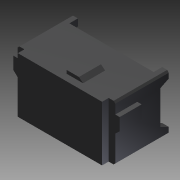
# Autodesk Inventor part: AS11CHright12
Saved by Autodesk Inventor 2011 SP1 (Build 150282100, 282)
## iProperties
Created: 2018-06-01
Part Number: AS11CHright12
Catalog Web Link: www.cadenas.de
Description: AS - Series - Body 1_2 for Poles 1 - Right Angle-
Vendor: NKKSWITCHES
Document SubType Name: Modeling
Designer: psAdmin
Manufacturer: NKKSWITCHES
Mass: 0.217145 g
Surface Area: 2.37031 cm^2
Volume: 0.217145 cm^3
Density: 1 g/cm^3
Category: PARTsolutions
Company: NKKSWITCHES
Title: AS11CHright12
Author: Cadenas PARTsolutions
PSOL_IDENT_0: {$CADENAS_DATA\23d-libs\nkkswitches\slides\as\parts\as_body_right1_2.prj},231 {VTYP=3D},{NB=AS11CHri
PSOL_IDENT_1: ght12},{LINA=AS11CHright12},{NN=AS - Series - Body 1_2 for Poles 1 - Right Angle},{DATE=11.10.2017 1
PSOL_IDENT_2: 0:53:50},{GEOMDATE=16.12.2008 13:32:00},{VERSION=},{LINEID=10},{LINESUBID=-1},{WBVAR=PLS,CRCTS,ACTU,
PSOL_IDENT_3: TRMNLS}  {NB=AS11CHright12},{LINA=AS11CHright12},{KT=DUMMY},{PN=AS11CH},{SRS=AS},{PLS=1},{CRCTS=1},{
PSOL_IDENT_4: ACTU=C},{TRMNLS=H},{CRCTSALG=  '1', '1 - ON/NONE/OFF','2', '2 - ON/NONE/ON', '3', '3 - ON/OFF/ON' }
NN: AS - Series - Body 1_2 for Poles 1 - Right Angle
NB: AS11CHright12
NBSYN: $PN.right12
LINA: AS11CHright12
PN: AS11CH
SRS: AS
PLS: 1 - SPST/SPDT
CRCTS: 1 - ON/NONE/OFF
ACTU: C - .150"(3,8mm)Long
TRMNLS: H - Right Angle with Bracket
SUPPLIER: NKKSWITCHES
ARTICLENO: AS11CHright12
BOMINFO: AS11CHright12
CREATOR: CADENAS GmbH
Autodesk Inventor part; units mm, degrees
sketch "Sketch_1" plane through (0, 0, 0) normal (0, 0, 1) x (1, 0, 0)
  line L0 (-4.4958, -2.3876) -> (-4.3434, -2.54)
  line L1 (-4.3434, -2.54) -> (4.3434, -2.54)
  line L2 (4.3434, -2.54) -> (4.4958, -2.3876)
  line L3 (4.4958, -2.3876) -> (4.4958, 2.3876)
  line L4 (4.4958, 2.3876) -> (4.3434, 2.54)
  line L5 (4.3434, 2.54) -> (-4.3434, 2.54)
  line L6 (-4.3434, 2.54) -> (-4.4958, 2.3876)
  line L7 (-4.4958, 2.3876) -> (-4.4958, -2.3876)
  constraints: 16 end point
extrude "Extrusion1" add sketch "Sketch_1" along normal blind 5.5499
sketch "Sketch_2" plane through (0, 0, 0) normal (0, 0, 1) x (1, 0, 0)
  line L0 (-3.8862, 2.54) -> (-3.8862, -2.54)
  line L1 (-3.8862, -2.54) -> (3.8862, -2.54)
  line L2 (3.8862, -2.54) -> (3.8862, 2.54)
  line L3 (3.8862, 2.54) -> (-3.8862, 2.54)
  constraints: 8 end point
extrude "Extrusion2" cut sketch "Sketch_2" along normal blind 0.7874
sketch "Sketch_14" plane through (0, 0, 0.7874) normal (0, 0, 1) x (1, 0, 0)
  line L0 (-3.8862, 2.413) -> (-3.8862, -2.413)
  line L1 (-3.8862, -2.413) -> (3.8862, -2.413)
  line L2 (3.8862, -2.413) -> (3.8862, 2.413)
  line L3 (3.8862, 2.413) -> (-3.8862, 2.413)
  constraints: 8 end point
extrude "Extrusion3" cut sketch "Sketch_14" along normal blind 0.0254
sketch "Sketch_3" plane through (4.4958, 0, 0) normal (1, 0, 0) x (0, 0, -1)
  line L0 (-0.7874, 1.5494) -> (-0.7874, -1.5494)
  line L1 (-0.7874, -1.5494) -> (0, -1.9304)
  line L2 (0, -1.9304) -> (0, 1.9304)
  line L3 (0, 1.9304) -> (-0.7874, 1.5494)
  constraints: 8 end point
extrude "Extrusion4" cut sketch "Sketch_3" against normal blind 8.9916
sketch "Sketch_4" plane through (0, 0, 4.9403) normal (0, 0, 1) x (1, 0, 0)
  line L0 (3.8862, 2.54) -> (3.8862, -2.54)
  line L1 (3.8862, -2.54) -> (4.4958, -2.54)
  line L2 (4.4958, -2.54) -> (4.4958, 2.54)
  line L3 (4.4958, 2.54) -> (3.8862, 2.54)
  constraints: 8 end point
extrude "Extrusion5" cut sketch "Sketch_4" along normal blind 0.6096
sketch "Sketch_5" plane through (0, 0, 4.9403) normal (0, 0, 1) x (1, 0, 0)
  line L0 (-4.4958, 2.54) -> (-4.4958, -2.54)
  line L1 (-4.4958, -2.54) -> (-3.8862, -2.54)
  line L2 (-3.8862, -2.54) -> (-3.8862, 2.54)
  line L3 (-3.8862, 2.54) -> (-4.4958, 2.54)
  constraints: 8 end point
extrude "Extrusion6" cut sketch "Sketch_5" along normal blind 0.6096
sketch "Sketch_6" plane through (0, 0, 4.9403) normal (0, 0, 1) x (1, 0, 0)
  line L0 (4.4958, 0) -> (4.9022, 0.381)
  line L1 (4.9022, 0.381) -> (4.9022, 1.524)
  line L2 (4.9022, 1.524) -> (4.4958, 1.524)
  line L3 (4.4958, 1.524) -> (4.4958, 0)
  constraints: 8 end point
extrude "Extrusion7" add sketch "Sketch_6" against normal blind 2.032
sketch "Sketch_7" plane through (0, 0, 4.9403) normal (0, 0, 1) x (1, 0, 0)
  line L0 (-4.9022, 0.381) -> (-4.4958, 0)
  line L1 (-4.4958, 0) -> (-4.4958, 1.524)
  line L2 (-4.4958, 1.524) -> (-4.9022, 1.524)
  line L3 (-4.9022, 1.524) -> (-4.9022, 0.381)
  constraints: 8 end point
extrude "Extrusion8" add sketch "Sketch_7" against normal blind 2.032
sketch "Sketch_8" plane through (0, 0, 4.9403) normal (0, 0, 1) x (1, 0, 0)
  line L0 (0, 2.8448) -> (0, 2.54)
  line L1 (0, 2.54) -> (1.524, 2.54)
  line L2 (1.524, 2.54) -> (1.143, 2.8448)
  line L3 (1.143, 2.8448) -> (0, 2.8448)
  constraints: 8 end point
extrude "Extrusion9" add sketch "Sketch_8" against normal blind 2.032
ref_plane "body1_right_XY" through (0, 0, 5.5499) normal (0, 0, -1) x (1, 0, 0)
ref_plane "body1_right_YZ" through (0, 0, 5.5499) normal (1, 0, 0) x (0, -1, 0)
ref_plane "body1_right_ZX" through (0, 0, 5.5499) normal (0, -1, 0) x (0, 0, -1)
ref_plane "cp_bracker_right_XY" through (0, -2.54, 4.9403) normal (0, 1, 0) x (1, 0, 0)
ref_plane "cp_bracker_right_YZ" through (0, -2.54, 4.9403) normal (1, 0, 0) x (0, 0, -1)
ref_plane "cp_bracker_right_ZX" through (0, -2.54, 4.9403) normal (0, 0, -1) x (0, 1, 0)
ref_plane "dummy_right_XY" through (-4.4958, -2.54, 0) normal (0, 1, 0) x (1, 0, 0)
ref_plane "dummy_right_YZ" through (-4.4958, -2.54, 0) normal (1, 0, 0) x (0, 0, -1)
ref_plane "dummy_right_ZX" through (-4.4958, -2.54, 0) normal (0, 0, -1) x (0, 1, 0)
ref_plane "terminal_h_XY" through (0, 0, 0.8636) normal (0, 0, 1) x (1, 0, 0)
ref_plane "terminal_h_YZ" through (0, 0, 0.8636) normal (1, 0, 0) x (0, 1, 0)
ref_plane "terminal_h_ZX" through (0, 0, 0.8636) normal (0, 1, 0) x (0, 0, 1)
body "Solid1"
